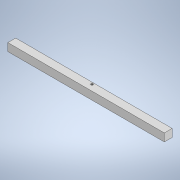
# Autodesk Inventor part: Piston_
Saved by Autodesk Inventor 2021 (Build 250183000, 183)
## iProperties
Created: 2022-06-12
Part Number: Piston_
Material: Generic
Document SubType Name: Modeling
Designer: authe
Density: 1 g/cm^3
Appearance: Default
Author: authe
Autodesk Inventor part; units mm, degrees
ref_plane "YZ Plane" through (0, 0, 0) normal (1, 0, 0) x (0, 1, 0)
ref_plane "XZ Plane" through (0, 0, 0) normal (0, 1, 0) x (-1, 0, 0)
ref_plane "XY Plane" through (0, 0, 0) normal (0, 0, 1) x (1, 0, 0)
sketch "Sketch1" plane through (0, 0, 0) normal (1, 0, 0) x (0, 1, 0)
  line L0 (0, 0) -> (30, 0)
  line L1 (30, 0) -> (30, -30)
  line L2 (30, -30) -> (0, -30)
  line L3 (0, -30) -> (0, 0)
  dimension "d0" = 30
  dimension "d1" = 30
  constraints: 8 end point, 2 parallel, 1 horizontal, 1 perpendicular
  measures "d0" distance of L0.start L0.end
  measures "d1" distance of L0.end L1.end
extrude "Extrusion1" add sketch "Sketch1" along normal blind 600
sketch "Sketch2" plane through (0, 30, 0) normal (0, 1, 0) x (1, 0, 0)
  circle A0 centre (300, 22.5) radius 4
  line L0 (0, 0) -> (600, 0) projected
  line L1 (0, 30) -> (0, 0) projected
  line L2 (600, 30) -> (600, 0) projected
  dimension "d4" = 8
  dimension "d5" = 22.5
  dimension "d6" = 300
  dimension "d7" = 600
  constraints: 1 centre point
  measures "d4" diameter of A0
  measures "d5" distance from line of L0 A0.centre
  measures "d6" distance from line of L1 A0.centre
  measures "d7" distance between parallel lines of L1 L2
extrude "Extrusion2" cut sketch "Sketch2" against normal through all
thread "Thread1" size "TR8x1.5" class "7H" standard "ISO Metric Trapezoidal Threads" full length
equation "\"d6\" = 0.5 * d7"
body "Solid1"
